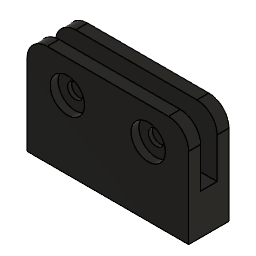
Apoyo pared lateral (Autodesk Fusion 360 design; units mm, degrees)
Autodesk Fusion 360 part; units mm, degrees
note: some values were not read from the file. Set by a fixed rule: which sketch regions a step uses.
sketch "Boceto1" plane through (0, 0, 0) normal (0, 1, 0) x (1, 0, 0)
  line L0 (0, 0) -> (40, 0)
  line L1 (40, 0) -> (40, -25)
  line L2 (40, -25) -> (0, -25)
  line L3 (0, -25) -> (0, 0)
  line L4 (20, 0) -> (20, -17)
  line L5 (20, -17) -> (10, -17)
  line L6 (20, -17) -> (30, -17)
  circle A0 centre (10, -17) radius 1.9
  circle A1 centre (30, -17) radius 1.9
  line L7 (40, 0) -> (0, 0)
  line L8 (0, 0) -> (0, -10)
  line L9 (0, -10) -> (40, -10)
  line L10 (40, -10) -> (40, 0)
  dimension "d1" = 40
  dimension "d2" = 25
  dimension "d3" = 3.8
  dimension "d4" = 3.8
  dimension "d5" = 10
  constraint horizontal L0
  constraint vertical L1
  constraint horizontal L2
  constraint vertical L3
  constraint coincident L0.start L3.end
  constraint midpoint L0 L4.start
  constraint perpendicular L0 L4
  constraint perpendicular L4 L5
  constraint perpendicular L4 L6
  constraint coincident L5.end A0.centre
  constraint coincident L6.end A1.centre
  constraint horizontal L7
  constraint vertical L8
  constraint horizontal L9
  constraint vertical L10
  measures "d1" distance of L0.start L0.end
  measures "d2" distance of L0.start L2.end
  measures "d3" diameter of A0
  measures "d4" diameter of A1
  measures "d5" distance of L0.end L9.end
extrude "Extruir1" add sketch "Boceto1" along normal blind 10 makes body 1
copy_body "Cuerpo - > Comp.1" bodies 1 removing the originals makes body 2 in component "Apoyo pared lateral"
extrude "Extruir1'" cut sketch "Boceto1" along normal blind 7 contours L1 L2 L3 L9 bodies 2 in component "Apoyo pared lateral"
extrude "Extruir2" add sketch "Boceto1" along normal blind 3 contours L1 L2 L3 L9 bodies 2 in component "Apoyo pared lateral"
fillet "Empalme1" radius 5 4 edges at (0, 1.5, 25) (0, 8.5, 25) (40, 1.5, 25) (40, 8.5, 25) on bodies 2 in component "Apoyo pared lateral"
move_face "CarasDesfase1" offset -0.05 2 faces at (16.9833, 7, 22.8818) (16.9833, 3, 22.8818) on bodies 2 in component "Apoyo pared lateral"
sketch "Boceto2" plane through (0, 0, 0) normal (0, -1, 0) x (1, 0, 0)
  arc A0 (40, 20) -> (35, 25) centre (35, 20) ccw
  line L0 (35, 25) -> (5, 25)
  arc A1 (5, 25) -> (0, 20) centre (5, 20) ccw
  line L1 (0, 20) -> (0, 0)
  line L2 (0, 0) -> (40, 0)
  line L3 (40, 0) -> (40, 20)
  circle A2 centre (30, 17) radius 1.9
  circle A3 centre (10, 17) radius 1.9
  circle A4 centre (10, 17) radius 3.5
  circle A5 centre (30, 17) radius 3.5
  dimension "d15" = 7
  dimension "d16" = 7
  constraint concentric A3 A4
  constraint concentric A2 A5
  measures "d15" diameter of A4
  measures "d16" diameter of A5
extrude "Extruir3" cut sketch "Boceto2" against normal blind 1.75 contours A4 | A5 bodies 2 in component "Apoyo pared lateral"
sketch "Boceto3" plane through (0, 10, 0) normal (0, 1, 0) x (-1, 0, 0)
  arc A0 (-35, 25) -> (-40, 20) centre (-35, 20) ccw
  line L0 (-40, 20) -> (-40, 0)
  line L1 (-40, 0) -> (0, 0)
  line L2 (0, 0) -> (0, 20)
  arc A1 (0, 20) -> (-5, 25) centre (-5, 20) ccw
  line L3 (-5, 25) -> (-35, 25)
  circle A2 centre (-30, 17) radius 1.9
  circle A3 centre (-10, 17) radius 1.9
extrude "Extruir4" add sketch "Boceto3" against normal blind 1.75 contours A2 | A3 bodies 2 in component "Apoyo pared lateral"
move_face "CarasDesfase3" offset -0.75 2 faces at (13.4956, 0.5833, 16.8255) (33.4826, 1.1667, 16.6515) on bodies 2 in component "Apoyo pared lateral"
extrude "Extruir5" cut 2 faces at (33.4438, 1.75, 16.6945) (13.4438, 1.75, 16.6945) along direction (0, 1, 0) blind 0.2 on bodies 2 bodies 2 in component "Apoyo pared lateral"
extrude "Extruir6" cut 2 faces at (10.6052, 8.25, 17.1867) (30.6278, 8.25, 17.6539) along direction (0, 1, 0) blind 2 on bodies 2 bodies 2 in component "Apoyo pared lateral"
component "Apoyo pared lateral" placed x (1, 0, 0) y (0, 1, 0) z (0, 0, 1) at (0, 0, 0)
named bodies: "Apoyo pared lateral"
